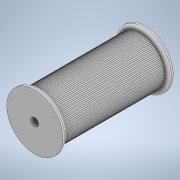
# Autodesk Inventor part: Trục băng chuyền
Saved by Autodesk Inventor 2020 (Build 240168000, 168)
## iProperties
Created: 2022-03-31
Part Number: Trục băng chuyền
Material: Generic
Document SubType Name: Modeling
Designer: PC
Density: 1 g/cm^3
Appearance: Default
Author: PC
Autodesk Inventor part; units mm, degrees
ref_plane "YZ Plane" through (0, 0, 0) normal (1, 0, 0) x (0, 1, 0)
ref_plane "XZ Plane" through (0, 0, 0) normal (0, 1, 0) x (-1, 0, 0)
ref_plane "XY Plane" through (0, 0, 0) normal (0, 0, 1) x (1, 0, 0)
sketch "Sketch1" plane through (0, 0, 0) normal (1, 0, 0) x (0, 1, 0)
  line L0 (0, 0) -> (0, -11.3344)
  line L1 (4.05, 0) -> (29.05, 0)
  line L2 (29.05, 0) -> (29.05, -5)
  line L3 (29.05, -5) -> (4.05, -5)
  line L4 (4.05, -5) -> (4.05, 0)
  line L5 (25.05, -5) -> (25.05, -110)
  line L6 (-4.05, -105) -> (-4.05, -110)
  line L7 (29.05, -110) -> (4.05, -110)
  line L8 (4.05, -110) -> (4.05, -115)
  line L9 (4.05, -115) -> (29.05, -115)
  line L10 (29.05, -115) -> (29.05, -110)
  line L11 (4.05, -5) -> (4.05, -110)
  point P0 (25.05, -110)
  dimension "d0" = 25
  dimension "d1" = 5
  dimension "d2" = 105
  dimension "d4" = 4
  dimension "d5" = 5
  dimension "d6" = 4.05
  dimension "d8" = 4.05
  dimension "d18" = 105
  constraints: 24 end point, 3 parallel, 3 perpendicular, 3 vertical, 2 horizontal, 1 point on line
  measures "d0" distance of L1.start L1.end
  measures "d1" distance of L1.end L2.end
  measures "d2" distance of L5.start L5.end
  measures "d4" distance between parallel lines of L2 L5
  measures "d5" distance of L6.end L6.start
  measures "d6" distance between parallel lines of L4 L0
  measures "d8" distance between parallel lines of L0 L6
  measures "d18" distance of L3.end L11.end
revolve "Revolution1" add sketch "Sketch1" angle 360 about axis through (0, 0, 0) along (0, 0, -1)
fillet "Fillet1" radius 3 2 edges at (0, -29.05, -110) (0, -29.05, -5)
sketch "Sketch2" plane through (0, 0, -5) normal (0, 0, -1) x (-1, 0, 0)
  circle A0 centre (0, 0) radius 25.05 projected
  circle A1 centre (0, 25.05) radius 0.75
  dimension "d11" = 1.5
  constraints: 1 centre point, 1 vertical alignment, 1 other
  measures "d11" diameter of A1
extrude "Extrusion1" cut sketch "Sketch2" along normal blind 105 contours A1 A0 | A0 A1 picked at (-0.0298, 24.801) picked at (0.0284, 25.2975)
pattern_circular "Circular Pattern1" count 60 over 360 about axis through (0, 0, -57.5) along (0, 0, -1) of "Extrusion1"
body "Solid1"
